Autodesk Fusion 360 part; units mm, degrees
(part 8 of 8)
  spline S2462 degree 3 poles (11.3202, -118.7507) (11.298, -118.7333) (11.2945, -118.7664) (11.3107, -118.8373) knots 0 0 0 0 1 1 1 1
  spline S2463 degree 3 poles (10.7859, -119.721) (10.7915, -119.7254) (10.8311, -119.7205) (10.8723, -119.7079) knots 0 0 0 0 1 1 1 1
  spline S2464 degree 3 poles (10.8723, -119.7079) (10.941, -119.6945) (10.9404, -119.6895) (10.8677, -119.6909) knots 0 0 0 0 1 1 1 1
  spline S2465 degree 3 poles (10.8677, -119.6909) (10.795, -119.6923) (10.7637, -119.7037) (10.7859, -119.721) knots 0 0 0 0 1 1 1 1
  spline S2466 degree 3 poles (10.9623, -119.7245) (10.9678, -119.7289) (11.0075, -119.724) (11.0486, -119.7114) knots 0 0 0 0 1 1 1 1
  spline S2467 degree 3 poles (11.0486, -119.7114) (11.1173, -119.6979) (11.1167, -119.693) (11.044, -119.6944) knots 0 0 0 0 1 1 1 1
  spline S2468 degree 3 poles (11.044, -119.6944) (10.9713, -119.6958) (10.94, -119.7071) (10.9623, -119.7245) knots 0 0 0 0 1 1 1 1
  spline S2469 degree 3 poles (11.3116, -119.8676) (11.3278, -119.9385) (11.3328, -119.9379) (11.3314, -119.8652) knots 0 0 0 0 1 1 1 1
  spline S2470 degree 3 poles (11.3314, -119.8652) (11.3315, -119.825) (11.3266, -119.7853) (11.3211, -119.781) knots 0 0 0 0 1 1 1 1
  spline S2471 degree 3 poles (11.3211, -119.781) (11.2988, -119.7636) (11.2953, -119.7967) (11.3116, -119.8676) knots 0 0 0 0 1 1 1 1
  spline S2472 degree 3 poles (11.3081, -120.044) (11.3244, -120.1149) (11.3293, -120.1142) (11.3279, -120.0415) knots 0 0 0 0 1 1 1 1
  spline S2473 degree 3 poles (11.3279, -120.0415) (11.328, -120.0013) (11.3231, -119.9617) (11.3176, -119.9574) knots 0 0 0 0 1 1 1 1
  spline S2474 degree 3 poles (11.3176, -119.9574) (11.2953, -119.94) (11.2919, -119.9731) (11.3081, -120.044) knots 0 0 0 0 1 1 1 1
  spline S2475 degree 3 poles (10.4202, -121.4096) (10.4365, -121.4805) (10.4414, -121.4799) (10.44, -121.4072) knots 0 0 0 0 1 1 1 1
  spline S2476 degree 3 poles (10.44, -121.4072) (10.4401, -121.367) (10.4353, -121.3273) (10.4297, -121.323) knots 0 0 0 0 1 1 1 1
  spline S2477 degree 3 poles (10.4297, -121.323) (10.4075, -121.3056) (10.404, -121.3387) (10.4202, -121.4096) knots 0 0 0 0 1 1 1 1
  spline S2478 degree 3 poles (11.309, -121.0743) (11.3252, -121.1452) (11.3302, -121.1446) (11.3288, -121.0719) knots 0 0 0 0 1 1 1 1
  spline S2479 degree 3 poles (11.3288, -121.0719) (11.3274, -120.9991) (11.316, -120.9679) (11.2986, -120.9901) knots 0 0 0 0 1 1 1 1
  spline S2480 degree 3 poles (11.2986, -120.9901) (11.2943, -120.9957) (11.2991, -121.0353) (11.309, -121.0743) knots 0 0 0 0 1 1 1 1
  spline S2481 degree 3 poles (10.8328, -122.3542) (10.8383, -122.3585) (10.8779, -122.3537) (10.9191, -122.3411) knots 0 0 0 0 1 1 1 1
  spline S2482 degree 3 poles (10.9191, -122.3411) (10.9878, -122.3276) (10.9872, -122.3227) (10.9145, -122.3241) knots 0 0 0 0 1 1 1 1
  spline S2483 degree 3 poles (10.9145, -122.3241) (10.8418, -122.3254) (10.8105, -122.3368) (10.8328, -122.3542) knots 0 0 0 0 1 1 1 1
sketch "Sketch20" plane through (0, 0, 0) normal (0, 1, 0) x (1, 0, 0)
  line L0 (6.9787, -102.7179) -> (6.9787, -125)
  line L1 (6.9787, -125) -> (9.0133, -126.4444)
  line L2 (9.0133, -126.4444) -> (10.24, -125.3374)
  line L3 (10.24, -125.3374) -> (11.3561, -124.3302)
  line L4 (11.3561, -124.3302) -> (11.3561, -123.7217)
  line L5 (11.3561, -123.7217) -> (12.6037, -122.1958)
  line L6 (12.6037, -122.1958) -> (11.9799, -120.8494)
  line L7 (11.9799, -120.8494) -> (11.7, -120)
  line L8 (11.7, -120) -> (11.9799, -119.6828)
  line L9 (11.9799, -119.6828) -> (12.7, -119.1)
  line L10 (12.7, -119.1) -> (12.7, -118.8667)
  line L11 (12.7, -118.8667) -> (11.9799, -117.6561)
  line L12 (11.9799, -117.6561) -> (12.8, -116.2)
  line L13 (12.8, -116.2) -> (11.8401, -114.4741)
  line L14 (11.8401, -114.4741) -> (12.0147, -113.5647)
  line L15 (12.0147, -113.5647) -> (13.1, -112.8)
  line L16 (13.1, -112.8) -> (13.0368, -111.695)
  line L17 (13.0368, -111.695) -> (12.5057, -110.7419)
  line L18 (12.5057, -110.7419) -> (12.3675, -109.727)
  line L19 (12.3675, -109.727) -> (12.7094, -109.4433)
  line L20 (12.7094, -109.4433) -> (13.05, -109.2)
  line L21 (13.05, -109.2) -> (13.0933, -109.1248)
  line L22 (13.0933, -109.1248) -> (13.0717, -109.0309)
  line L23 (13.0717, -109.0309) -> (12.4, -108)
  line L24 (12.4, -108) -> (12.4, -106.6)
  line L25 (12.4, -106.6) -> (13.2, -106.6)
  line L26 (13.2, -106.6) -> (13.2, -102.7)
  line L27 (13.2, -102.7) -> (13.7, -102.3)
  line L28 (13.7, -102.3) -> (14.8, -102.3)
  line L29 (14.8, -102.3) -> (15.9, -102)
  line L30 (15.9, -102) -> (16.8, -101.1)
  line L31 (16.8, -101.1) -> (17.1, -99.9)
  line L32 (17.1, -99.9) -> (17.1, -98)
  line L33 (17.1, -98) -> (17.1, -95.6)
  line L34 (17.1, -95.6) -> (17.1, -92.2)
  line L35 (17.1, -92.2) -> (17.1, -89.4)
  line L36 (17.1, -89.4) -> (16.7293, -88.5038)
  line L37 (16.7293, -88.5038) -> (15.7905, -87.6026)
  line L38 (15.7905, -87.6026) -> (14.8329, -87.4148)
  line L39 (14.8329, -87.4148) -> (5.0693, -87.5087)
  line L40 (5.0693, -87.5087) -> (4.1868, -87.7903)
  line L41 (4.1868, -87.7903) -> (3.3794, -88.5602)
  line L42 (3.3794, -88.5602) -> (3.0602, -89.7618)
  line L43 (3.0602, -89.7618) -> (3.0602, -100)
  line L44 (3.0602, -100) -> (3.3794, -101.2041)
  line L45 (3.3794, -101.2041) -> (4.1755, -101.865)
  line L46 (4.1755, -101.865) -> (6.3029, -102.2781)
  line L47 (6.3029, -102.2781) -> (6.9787, -102.7179)
  line L48 (9.4358, -126.0631) -> (9.3013, -104.6804)
  line L49 (9.3013, -104.6804) -> (10.3411, -104.6739)
  line L50 (10.3411, -104.6739) -> (10.3411, -125.2462)
  line L51 (11.3561, -123.7217) -> (11.3561, -104.6771)
  line L52 (11.3561, -104.6771) -> (13.2, -104.65)
  circle A0 centre (10, -91.5) radius 1.9557
  circle A1 centre (10, -91.5) radius 2.678
  constraint vertical L0
  constraint parallel L2 L3
  constraint vertical L4
  constraint vertical L10
  constraint vertical L24
  constraint perpendicular L24 L25
  constraint perpendicular L25 L26
  constraint perpendicular L26 L28
  constraint perpendicular L28 L32
  constraint parallel L32 L33
  constraint parallel L32 L34
  constraint parallel L34 L35
  constraint vertical L43
  constraint coincident L2 L48.start
  constraint perpendicular L48 L49
  constraint coincident L3 L50.end
  constraint vertical L50
  constraint parallel L50 L51
  constraint midpoint L26 L52.end
  constraint concentric A0 A1
extrude "Extrude12" add sketch "Sketch20" along normal blind 1.5 separate body contours L0 L1 L2 L3 L4 L26 L27 L28 L29 L30 L31 L32 L33 L34 L35 L36 L37 L38 L39 L40 L41 L42 L43 L44 L45 L46 L47 L48 L49 L50 L51 L52 makes body 9
extrude "Extrude13" cut 1 faces at (10.1263, 1.5, 99.8628) along direction (0, -1, 0) blind 1 on bodies 9 bodies 9
extrude "Extrude14" add sketch "Sketch19" against normal blind 0.5 contours S1226 S1227 S1228 S1229 S1230 S1231 S1232 S1233 S1234 S1235 S1236 S1237 S1238 S1239 S1240 S1241 S1242 S1243 S1244 S1245 S1246 S1247 S1248 S1249 S1250 S1251 S1252 S1253 S1254 S1255 S1256 S1257 S1258 S1259 S1260 S1261 S1262 S1263 S1264 S1265 S1266 S1267 S1268 S1269 S1270 S1271 S1272 S1273 S1274 S1275 S1276 S1277 S1278 S1279 S1280 S1281 S1282 S1283 S1284 S1285 S1286 S1287 S1288 S1289 S1290 S1291 S1292 S1293 S1294 S1295 S1296 S1297 S1298 S1299 S1300 S1301 S1302 S1303 S1304 S1305 S1306 S1307 S1308 S1309 S1310 S1311 S1312 S1313 S1314 S1315 S1316 S1317 S1318 S1319 S1320 S1321 S1322 S1323 S1324 S1325 S1326 S1327 S1328 S1329 S1330 S1331 S1332 S1333 S1334 S1335 S1336 S1337 S1338 S1339 S1340 S1341 S1342 S1343 S1344 S1345 L106 L107 S1346 S1347 S1348 S1349 S1350 S1351 S1352 S1353 S1354 S1355 S1356 S1357 S1358 L108 L109 L110 L111 S1359 S1360 S1361 S1362 S1363 S1364 S1365 S1366 S1367 S1368 S1369 S1370 S1371 S1372 S1373 S1374 S1375 S1376 S1377 S1378 S1379 S1380 S1381 S1382 S1383 S1384 S1385 S1386 S1387 S1388 S1389 S1390 S1391 S1392 S1393 S1394 S1395 S1396 S1397 S1398 S1399 S1400 S1401 S1402 S1403 S1404 S1405 S1406 S1407 S1408 S1409 S1410 S1411 S1412 S1413 S1414 S1415 | S1416 S1417 S1418 S1419 S1420 S1421 S1422 S1423 S1424 S1425 S1426 S1427 S1428 S1429 S1430 S1431 S1432 S1433 S1434 S1435 S1436 S1437 S1438 S1439 S1440 S1441 S1442 S1443 S1444 S1445 S1446 S1447 S1448 S1449 S1450 S1451 S1452 S1453 S1454 S1455 S1456 S1457 S1458 L112 L113 L114 L115 S1459 S1460 S1461 S1462 S1463 S1464 S1465 S1466 S1467 S1468 S1469 S1470 S1471 S1472 S1473 S1474 S1475 S1476 S1477 S1478 S1479 S1480 S1481 S1482 S1483 S1484 S1485 S1486 S1487 S1488 S1489 S1490 S1491 S1492 S1493 S1494 S1495 bodies 9
move_body "Move1" bodies 9 to x (-1, 0, 0) y (0, -1, 0) z (0, 0, 1) at (17.8327, 9.6069, -57.9853)
move_body "Move2" bodies 9 to x (1, 0, 0) y (0, 1, 0) z (0, 0, 1) at (-0.2462, 0.6485, -0.0308)
sketch "Sketch21" plane through (0, 0, 28.5) normal (0, 0, 1) x (-1, 0, 0)
  line L0 (-8.5, -11) -> (-8.5, -9)
  line L1 (-8.5, -9) -> (-6.5, -9)
  line L2 (-6.5, -9) -> (-6.5, -11)
  line L3 (-6.5, -11) -> (-8.5, -11)
  arc A0 (0, -3) -> (-3, 0) centre (-3, -3) ccw
  line L4 (-3, 0) -> (-12, 0)
  arc A1 (-12, 0) -> (-15, -3) centre (-12, -3) ccw
  line L5 (-15, -3) -> (-15, -17)
  arc A2 (-15, -17) -> (-12, -20) centre (-12, -17) ccw
  line L6 (-12, -20) -> (-3, -20)
  arc A3 (-3, -20) -> (0, -17) centre (-3, -17) ccw
  line L7 (0, -17) -> (0, -3)
  line L8 (-14.2, -10.3) -> (-13.5, -10.3)
  line L9 (-13.5, -10.3) -> (-13.5, -10.5)
  line L10 (-13.5, -10.5) -> (-14.2, -10.5)
  line L11 (-14.2, -10.5) -> (-14.2, -10.3)
  line L12 (-14.2, -9.7) -> (-13.5, -9.7)
  line L13 (-13.5, -9.7) -> (-13.5, -9.5)
  line L14 (-13.5, -9.5) -> (-14.2, -9.5)
  line L15 (-14.2, -9.5) -> (-14.2, -9.7)
  line L16 (-0.7, -10.3) -> (-1.4, -10.3)
  line L17 (-1.4, -10.3) -> (-1.4, -10.5)
  line L18 (-1.4, -10.5) -> (-0.7, -10.5)
  line L19 (-0.7, -10.5) -> (-0.7, -10.3)
  line L20 (-0.7, -9.7) -> (-1.4, -9.7)
  line L21 (-1.4, -9.7) -> (-1.4, -9.5)
  line L22 (-1.4, -9.5) -> (-0.7, -9.5)
  line L23 (-0.7, -9.5) -> (-0.7, -9.7)
  constraint horizontal L8
  constraint vertical L9
  constraint horizontal L10
  constraint vertical L11
  constraint horizontal L12
  constraint vertical L13
  constraint horizontal L14
  constraint vertical L15
  constraint horizontal L16
  constraint vertical L17
  constraint horizontal L18
  constraint vertical L19
  constraint horizontal L20
  constraint vertical L21
  constraint horizontal L22
  constraint vertical L23
extrude "Extrude15" add sketch "Sketch21" along normal blind 1.5 contours L8 L9 L10 L11 | L12 L13 L14 L15 | L16 L17 L18 L19 | L20 L21 L22 L23 bodies 2
move_body "Move3" bodies 9 to x (1, 0, 0) y (0, 1, 0) z (0, 0, 1) at (0, 0, -0.5)
copy_body "Body->Comp3" bodies 2 removing the originals makes body 10 in component "Basic_light"
copy_body "Body->Comp4" bodies 6 removing the originals makes body 11 in component "flash light"
copy_body "Body->Comp5" bodies 9 removing the originals makes body 12 in component "key"
component "buttons" placed x (1, 0, 0) y (0, 1, 0) z (0, 0, 1) at (0, 0, 0)
component "Dicoration part" placed x (1, 0, 0) y (0, 1, 0) z (0, 0, 1) at (-0.0272, -0.0097, 0.517)
component "body_function" placed x (1, 0, 0) y (0, 1, 0) z (0, 0, 1) at (0, 0, 0)
component "Basic_light" placed x (1, 0, 0) y (0, 1, 0) z (0, 0, 1) at (0, 0, 0)
component "flash light" placed x (1, 0, 0) y (0, 1, 0) z (0, 0, 1) at (0, 0, 0)
component "key" placed x (1, 0, 0) y (0, 1, 0) z (0, 0, 1) at (0, 0, 0)
named bodies: "Dicoration part", "Basic_light", "body_function", "flash light", "key"
